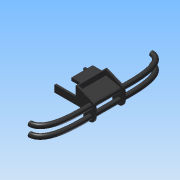
# Autodesk Inventor part: FrontBumper
Saved by Autodesk Inventor 2014 (Build 180170000, 170)
## iProperties
Created: 2014-01-01
Part Number: FrontBumper
Material: ABS Plastic
Document SubType Name: Modeling
Designer: davidgitz
Density: 1 g/cm^3
Appearance: Dark Gray
Author: davidgitz
Autodesk Inventor part; units mm, degrees
ref_plane "YZ Plane" through (0, 0, 0) normal (1, 0, 0) x (0, 1, 0)
sketch "Sketch1" plane through (0, 0, 0) normal (0, 0, 1) x (1, 0, 0)
  circle A0 centre (0.0168, -0.8888) radius 5.334
  circle A1 centre (0.0168, 19.9392) radius 5.334
  line L0 (0.0168, 19.9392) -> (0.0168, -0.8888) construction
  point P0 (0, 0)
  dimension "d0" = 10.668
  dimension "d3" = 10.16
  constraints: 2 centre point, 2 end point, 1 equal radius, 1 vertical
  measures "d0" diameter of A0
extrude "Extrusion1" add sketch "Sketch1" along normal mid plane 60.96
sketch "Sketch2" plane through (0.0168, 19.9392, 30.48) normal (0, 0, 1) x (1, 0, 0)
  circle A0 centre (0, 0) radius 5.334 projected
  arc A1 (10.414, 0) -> (3.9458, 9.6376) centre (0, 0) ccw
  line L0 (-29.591, 23.368) -> (3.9458, 9.6376)
  line L1 (10.414, 0) -> (10.414, -20.828)
  arc A2 (0, -31.242) -> (10.414, -20.828) centre (0, -20.828) ccw
  line L2 (-29.591, 23.368) -> (-29.591, 1.143)
  line L3 (-29.591, 1.143) -> (-79.756, 1.143)
  line L4 (-79.756, 1.143) -> (-79.756, -14.097)
  line L5 (-79.756, -14.097) -> (-14.986, -14.097)
  line L6 (-14.986, -14.097) -> (-14.986, -31.242)
  line L7 (-14.986, -31.242) -> (0, -31.242)
  line L8 (5.334, 21.0773) -> (5.334, -9.8858) construction
  circle A3 centre (0, -20.828) radius 5.334 construction
  line L9 (-9.5742, -26.162) -> (14.8668, -26.162) construction
  point P0 (-0.0168, -19.9392)
  point P1 (-0.4616, -10.4242)
  dimension "d4" = 5.08
  dimension "d6" = 22.225
  dimension "d7" = 15.24
  dimension "d8" = 17.145
  dimension "d9" = 5.08
  dimension "d10" = 50.165
  dimension "d11" = 40.005
  dimension "d12" = 90.17
  dimension "d13" = 25.4
  constraints: 20 end point, 5 point on circle, 5 tangent, 4 parallel, 3 perpendicular, 2 centre point, 1 coincident, 1 concentric, 1 horizontal, 1 vertical
  measures "d4" distance between parallel lines of L8 L1
  measures "d6" distance of L0.start L2.end
  measures "d7" distance of L3.end L4.end
  measures "d8" distance between parallel lines of L7 L5
  measures "d9" distance between parallel lines of L7 L9
  measures "d10" distance between parallel lines of L4 L2
  measures "d11" distance between parallel lines of L1 L2
  measures "d12" distance between parallel lines of L1 L4
  measures "d13" distance between parallel lines of L1 L6
extrude "Extrusion2" add sketch "Sketch2" along normal blind 4.064 contours A0 | L1 A2 L7 L6 L5 L4 L3 L2 L0 A1
mirror "Mirror1" about plane through (0, 0, 0) normal (0, 0, 1) of "Extrusion2"
sketch "Sketch3" plane through (-29.5742, 21.0822, 30.48) normal (-1, 0, 0) x (0, 0, 1)
  line L0 (4.064, 22.225) -> (-65.024, 22.225)
  line L1 (-65.024, 22.225) -> (-65.024, 0)
  line L2 (-65.024, 0) -> (4.064, 0)
  line L3 (4.064, 0) -> (4.064, 22.225)
  line L4 (-60.96, -1.143) -> (-65.024, -1.143) projected
  line L5 (-65.024, -1.143) -> (-65.024, 8.4946) projected
  line L6 (-65.024, 8.4946) -> (-65.024, 22.225) projected
  line L7 (-65.024, -1.143) -> (-65.024, 8.4946) projected
  line L8 (-65.024, -21.971) -> (-65.024, -1.143) projected
  line L9 (-65.024, -32.385) -> (-65.024, -21.971) projected
  line L10 (-65.024, -15.24) -> (-65.024, -32.385) projected
  line L11 (-65.024, 0) -> (-65.024, -15.24) projected
  line L12 (-65.024, 22.225) -> (-65.024, 0) projected
  line L13 (-60.96, 0) -> (-65.024, 0) projected
  point P0 (-30.48, -21.0822)
  constraints: 8 end point, 2 parallel, 1 horizontal, 1 perpendicular
extrude "Extrusion3" add sketch "Sketch3" along normal blind 2.54
sketch "Sketch4" plane through (0.0168, 19.9392, 30.48) normal (0, 0, -1) x (-1, 0, 0)
  circle A0 centre (0, 0) radius 5.334 projected
  arc A1 (-3.9458, 9.6376) -> (-10.414, 0) centre (0, 0) ccw projected
  line L0 (29.591, 1.143) -> (29.591, 23.368) projected
  line L1 (-2.8511, 4.8505) -> (29.591, 11.684)
  arc A2 (3.8702, 3.6705) -> (-1.0994, 5.2195) centre (0, 0) ccw
  line L2 (3.8702, 3.6705) -> (29.591, 9.0883)
  line L3 (29.591, 11.684) -> (29.591, 9.0883)
  point P0 (0.0168, -19.9392)
  dimension "d18" = 2.54
  dimension "d22" = 11.684
  constraints: 6 end point, 3 point on line, 2 point on circle, 1 centre point, 1 coincident, 1 collinear, 1 concentric, 1 parallel, 1 tangent
  measures "d18" distance between parallel lines of L2 L1
  measures "d22" distance of L0.end L1.end
extrude "Extrusion4" add sketch "Sketch4" along normal up to next contours A0 L1 L0 L2
sketch "Sketch5" plane through (0.0168, 19.9392, 34.544) normal (0, 0, 1) x (1, 0, 0)
  arc A0 (0, -31.242) -> (10.414, -20.828) centre (0, -20.828) ccw projected
  circle A1 centre (0, -20.828) radius 5.334 projected
  point P0 (-0.0168, -19.9392)
ref_plane "Work Plane1" through (0.0168, -0.8888, 34.544) normal (0, 1, 0) x (0, 0, 1)
sketch "Sketch6" plane through (0.0168, -0.8888, 34.544) normal (0, 1, 0) x (0, 0, 1)
  line L0 (0, 0) -> (101.6, 0) construction
  line L1 (89.3192, 0) -> (89.3192, -12.7) construction
  line L2 (101.6, 0) -> (101.6, -32.766) construction
  spline S0 degree 2 poles (0, 0) (100.1002, 3.7047) (101.6, -32.766) knots 0 0 0 1 1 1
  line L3 (71.1265, 0) -> (71.1265, -5.0653) construction
  line L4 (-4.064, 10.414) -> (0, 10.414) projected
  point P0 (-34.544, -0.0168)
  point P1 (0, 0)
  dimension "d25" = 101.6
  dimension "d28" = 12.2808
  dimension "d29" = 30.4735
  dimension "d30" = 12.7
  dimension "d43" = 43.18
  constraints: 8 end point, 2 parallel, 2 point on line, 1 coincident, 1 horizontal, 1 perpendicular, 4 other
  measures "d25" horizontal distance of point (0, 0) L2.end
  measures "d28" distance between parallel lines of L1 L2
  measures "d29" distance between parallel lines of L3 L2
  measures "d30" distance from line of L1.end L0
  measures "d43" distance from line of L2.end L4
sweep "Sweep1" add profiles "Sketch5" path "Sketch6" path curves S0
sketch "Sketch7" plane through (0.0168, 19.9392, 34.544) normal (0, 0, 1) x (1, 0, 0)
  arc A0 (10.414, 0) -> (3.9458, 9.6376) centre (0, 0) ccw projected
  arc A1 (-3.8702, 3.6705) -> (1.0994, 5.2195) centre (0, 0) ccw projected
  circle A2 centre (0, 0) radius 5.334
  point P0 (5.334, -20.828)
  point P1 (-0.0168, -19.9392)
  constraints: 1 centre point, 1 coincident, 1 concentric
ref_plane "Work Plane2" through (0.0168, 19.9392, 34.544) normal (0, 1, 0) x (0, 0, 1)
sketch "Sketch8" plane through (0.0168, 19.9392, 34.544) normal (0, 1, 0) x (0, 0, 1)
  line L0 (0, 0) -> (101.6, 0) construction
  line L1 (89.3192, 0) -> (89.3192, -12.7) construction
  line L2 (101.6, 0) -> (101.6, -32.766) construction
  spline S0 degree 2 poles (0, 0) (100.1002, 3.7047) (101.6, -32.766) knots 0 0 0 1 1 1
  line L3 (71.1265, 0) -> (71.1265, -5.0653) construction
  line L4 (-104.9231, 0) -> (145.9225, 0) projected
  line L5 (0, 3.9458) -> (0, -29.591) projected
  line L6 (-4.064, 10.414) -> (0, 10.414) projected
  point P0 (-34.544, -0.0168)
  dimension "d31" = 101.6
  dimension "d33" = 12.2808
  dimension "d34" = 30.4735
  dimension "d35" = 12.7
  dimension "d44" = 43.18
  constraints: 8 end point, 4 point on line, 2 parallel, 1 coincident, 1 horizontal, 1 perpendicular, 4 other
  measures "d31" horizontal distance of point (0, 0) L2.end
  measures "d33" distance between parallel lines of L1 L2
  measures "d34" distance between parallel lines of L3 L2
  measures "d35" distance from line of L1.end L0
  measures "d44" distance from line of L2.end L6
sweep "Sweep2" add profiles "Sketch7" path "Sketch8" path curves S0
mirror "Mirror3" about plane through (0, 0, 0) normal (0, 0, 1) of "Sweep1", "Sweep2"
sketch "Sketch9" plane through (-32.1142, 21.0822, 30.48) normal (-1, 0, 0) x (0, 0, 1)
  line L0 (4.064, 22.225) -> (-65.024, 22.225) projected
  line L1 (-65.024, 22.225) -> (-65.024, 0) projected
  line L2 (-60.96, 0) -> (0, 0) projected
  line L3 (-30.48, 22.225) -> (-30.48, 0) construction
  line L4 (-54.356, 15.621) -> (-54.356, 22.225)
  line L5 (-54.356, 15.621) -> (-51.816, 15.621)
  line L6 (-51.816, 15.621) -> (-51.816, 19.685)
  line L7 (-51.816, 19.685) -> (-30.48, 19.685)
  line L8 (-54.356, 22.225) -> (-30.48, 22.225)
  line L9 (-6.604, 15.621) -> (-6.604, 22.225)
  line L10 (-6.604, 15.621) -> (-9.144, 15.621)
  line L11 (-9.144, 15.621) -> (-9.144, 19.685)
  line L12 (-9.144, 19.685) -> (-30.48, 19.685)
  line L13 (-6.604, 22.225) -> (-30.48, 22.225)
  point P0 (-30.48, -21.0822)
  dimension "d37" = 10.668
  dimension "d38" = 6.604
  dimension "d39" = 2.54
  dimension "d40" = 2.54
  constraints: 22 end point, 4 perpendicular, 4 symmetric about line, 2 midpoint, 2 point on line, 1 collinear
  measures "d37" distance between parallel lines of L1 L4
  measures "d38" distance of L4.start L4.end
  measures "d39" distance between parallel lines of L4 L6
  measures "d40" distance between parallel lines of L7 L8
extrude "Extrusion5" add sketch "Sketch9" along normal blind 20.32
body "Solid1"
